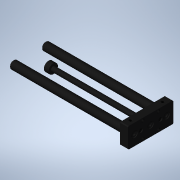
# Autodesk Inventor part: 170831 DFM-12-100-P-A-GF---(K)
Saved by Autodesk Inventor 2021 (Build 250183000, 183)
## iProperties
Created: 2025-06-15
Part Number: 170831 DFM-12-100-P-A-GF---(K)
Material: Generic
Catalog Web Link: www.cadenas.de
Description: DFM-(K)-Guide unit
Vendor: FESTO
Document SubType Name: Modeling
Designer: psAdmin
Manufacturer: FESTO
Mass: 40.9648 g
Surface Area: 173.4 cm^2
Volume: 40.9648 cm^3
Density: 1 g/cm^3
Appearance: PSOLRGB-128-128-128
Category: PARTsolutions
Company: FESTO
Title: 170831 DFM-12-100-P-A-GF---(K)
Author: Cadenas PARTsolutions
Comments: Guide unit
PSOL_IDENT_0: {$CADENAS_DATA/23d-libs/festo_fdt/parts/d/dfm/parts/dfm_k.prj},201 {VTYP=3D},{NB=170831 DFM-12-100-P
PSOL_IDENT_1: -A-GF---(K)},{LINA=170831 DFM-12-100-P-A-GF---(K)},{NN=DFM-(K)},{DATE=15.05.2025 16:58:02},{GEOMDATE=
PSOL_IDENT_2: 22.08.2023 11:13:07},{VERSION=},{LINEID=80},{WBVAR=},{WBNUMERIC=}  {NB=170831 DFM-12-100-P-A-GF---(K
PSOL_IDENT_3: )},{LINA=170831 DFM-12-100-P-A-GF---(K)},{KT=1},{TNR=170831},{TYP=DFM},{KDM=12},{HUB=100},{F=GF},{BW
PSOL_IDENT_4: E=-},{BWET=},{B4=30.000},{H1=28.000},{L8=21.000},{L9=40.000},{L11=80.000},{L7=6.000},{L1=155.000},{B
PSOL_IDENT_5: 1=60.000},{B2=58.000},{B3=42.400},{B5=4.500},{B6=51.000},{B7=20.500},{B8=19.000},{B9=20.000},{B10=20
PSOL_IDENT_6: .000},{B11=9.500},{B12=41.000},{B13=19.500},{B14=21.000},{D1=M 5},{D1P=5.000},{D1KDR=4.134},{D2=8.00
PSOL_IDENT_7: 0},{D3=9.000},{D4=M 4},{D4P=4.000},{D4KDR=3.242},{D5=0.000},{D6=M 4},{D6P=4.000},{D6KDR=3.242},{D7=1
PSOL_IDENT_8: 0},{D7GF=10.000},{D7KF=8.000},{D8=5.000},{FN=1},{FT=GF},{EE=M 5},{EEMM=5.000},{EEKDR=4.134},{H2=26.0
PSOL_IDENT_9: 00},{H3=24.000},{H4=14.000},{H5=14.000},{H6=4.000},{H7=20.000},{H8=0.000},{H9=4.000},{H10=20.000},{H
PSOL_IDENT_10: 11=14.000},{L2=136.000},{L3=10.000},{L4=13.000},{L5=11.400},{L6=9.500},{L10=34.000},{L12=11.400},{T1=
PSOL_IDENT_11: 9.000},{T2=9.400},{T3=2.100},{T4=8.000},{T5=0.000},{T6=1.000},{SW1=10.000},{SW1T=3.200},{SW2=10.000}
PSOL_IDENT_12: ,{SW2D=6.000},{SW2T=3.200},{ZZ=0},{MOD=1},{BR=8.000},{I1=25.000},{I2=41.000},{I3=4.000},{I4=8.000},{
PSOL_IDENT_13: DIML7=1},{YSCREW=0}
NB: 170831 DFM-12-100-P-A-GF---(K)
NN: DFM-(K)
NT: Guide unit
NBSYN: $TNR. $TYP.-$KDM.-$HUB.-P-A-$FT.$BWET.---(K)
LINA: 170831 DFM-12-100-P-A-GF---(K)
CATALOG: Festo Design Tool 3D
TNR: 170831
TYP: DFM
KDM: 12
HUB: 100
F: GF
BWE: -
B4: 30
H1: 28
L8: 21
L9: 40
L11: 80
L7: 6
L1: 155
B1: 60
B2: 58
B3: 42.4
B5: 4.5
B6: 51
B7: 20.5
B8: 19
B9: 20
B10: 20
B11: 9.5
B12: 41
B13: 19.5
B14: 21
D1: M 5
D1P: 5
D1KDR: 4.134
D2: 8
D3: 9
D4: M 4
D4P: 4
D4KDR: 3.242
D5: 0
D6: M 4
D6P: 4
D6KDR: 3.242
D7GF: 10
D7KF: 8
D8: 5
EE: M 5
EEKDR: 4.134
H2: 26
H3: 24
H4: 14
H5: 14
H6: 4
H7: 20
H8: 0
H9: 4
H10: 20
H11: 14
L2: 136
L3: 10
L4: 13
L5: 11.4
L6: 9.5
L10: 34
L12: 11.4
T1: 9
T2: 9.4
T3: 2.1
T4: 8
T5: 0
T6: 1
SW1: 10
SW1T: 3.2
SW2: 10
SW2D: 6
SW2T: 3.2
BR: 8
I1: 25
I2: 41
I3: 4
I4: 8
SUPPLIER: FESTO
ARTICLENO: 170831 DFM-12-100-P-A-GF---(K)
BOMINFO: 170831 DFM-12-100-P-A-GF---(K)
CREATOR: CADENAS GmbH
Autodesk Inventor part; units mm, degrees
ref_plane "YZ Plane" through (0, 0, 0) normal (1, 0, 0) x (0, 1, 0)
ref_plane "XZ Plane" through (0, 0, 0) normal (0, 1, 0) x (-1, 0, 0)
ref_plane "XY Plane" through (0, 0, 0) normal (0, 0, 1) x (1, 0, 0)
sketch "Sketch_2" plane through (13, 0, 0) normal (1, 0, 0) x (0, 0, -1)
  line L0 (-29, -12) -> (-28, -13)
  line L1 (-28, -13) -> (28, -13)
  line L2 (28, -13) -> (29, -12)
  line L3 (29, -12) -> (29, 12)
  line L4 (29, 12) -> (28, 13)
  line L5 (28, 13) -> (-28, 13)
  line L6 (-28, 13) -> (-29, 12)
  line L7 (-29, 12) -> (-29, -12)
  constraints: 16 end point
sketch "Sketch_3" plane through (0, 0, 0) normal (0, 1, 0) x (1, 0, 0)
  line L0 (13, 20.5) -> (-142, 20.5)
  line L1 (-142, 20.5) -> (-142, 24.5)
  line L2 (-142, 24.5) -> (-141, 25.5)
  line L3 (-141, 25.5) -> (13, 25.5)
  line L4 (13, 25.5) -> (13, 20.5)
  line L5 (13, 20.5) -> (-142, 20.5)
  constraints: 12 end point
sketch "Sketch_4" plane through (0, 0, 0) normal (0, 1, 0) x (1, 0, 0)
  line L0 (13, -20.5) -> (-142, -20.5)
  line L1 (-142, -20.5) -> (-142, -16.5)
  line L2 (-142, -16.5) -> (-141, -15.5)
  line L3 (-141, -15.5) -> (13, -15.5)
  line L4 (13, -15.5) -> (13, -20.5)
  line L5 (13, -20.5) -> (-142, -20.5)
  constraints: 12 end point
extrude "Extrusion1" add sketch "Sketch_2" against normal blind 10
sketch "Sketch_8" plane through (0, 10, 0) normal (0, 1, 0) x (1, 0, 0)
  line L0 (13, 10) -> (3, 10)
  line L1 (3, 10) -> (3, 12)
  line L2 (3, 12) -> (3.379, 11.621)
  line L3 (3.379, 11.621) -> (12.621, 11.621)
  line L4 (12.621, 11.621) -> (13, 12)
  line L5 (13, 12) -> (13, 10)
  line L6 (13, 10) -> (3, 10)
  constraints: 14 end point
revolve "Revolution1" cut sketch "Sketch_8" angle 360 about axis through (13, 10, -10) along (-1, 0, 0)
thread "Thread1" size "M4x0.7" class "6H" standard "ISO Metric profile" full length
sketch "Sketch_9" plane through (0, 10, 0) normal (0, 1, 0) x (1, 0, 0)
  line L0 (13, -10) -> (3, -10)
  line L1 (3, -10) -> (3, -8)
  line L2 (3, -8) -> (3.379, -8.379)
  line L3 (3.379, -8.379) -> (12.621, -8.379)
  line L4 (12.621, -8.379) -> (13, -8)
  line L5 (13, -8) -> (13, -10)
  line L6 (13, -10) -> (3, -10)
  constraints: 14 end point
revolve "Revolution2" cut sketch "Sketch_9" angle 360 about axis through (13, 10, 10) along (-1, 0, 0)
thread "Thread2" size "M4x0.7" class "6H" standard "ISO Metric profile" full length
sketch "Sketch_12" plane through (0, -10, 0) normal (0, 1, 0) x (1, 0, 0)
  line L0 (13, 10) -> (3, 10)
  line L1 (3, 10) -> (3, 12)
  line L2 (3, 12) -> (3.379, 11.621)
  line L3 (3.379, 11.621) -> (12.621, 11.621)
  line L4 (12.621, 11.621) -> (13, 12)
  line L5 (13, 12) -> (13, 10)
  line L6 (13, 10) -> (3, 10)
  constraints: 14 end point
revolve "Revolution3" cut sketch "Sketch_12" angle 360 about axis through (13, -10, -10) along (-1, 0, 0)
thread "Thread3" size "M4x0.7" class "6H" standard "ISO Metric profile" full length
sketch "Sketch_13" plane through (0, -10, 0) normal (0, 1, 0) x (1, 0, 0)
  line L0 (13, -10) -> (3, -10)
  line L1 (3, -10) -> (3, -8)
  line L2 (3, -8) -> (3.379, -8.379)
  line L3 (3.379, -8.379) -> (12.621, -8.379)
  line L4 (12.621, -8.379) -> (13, -8)
  line L5 (13, -8) -> (13, -10)
  line L6 (13, -10) -> (3, -10)
  constraints: 14 end point
revolve "Revolution4" cut sketch "Sketch_13" angle 360 about axis through (13, -10, 10) along (-1, 0, 0)
thread "Thread4" size "M4x0.7" class "6H" standard "ISO Metric profile" full length
sketch "Skizze_3" plane through (0, 0, 0) normal (0, 0, 1) x (1, 0, 0)
  line L0 (3, 0) -> (-117.4, 0)
  line L1 (-117.4, 0) -> (-117.4, 6)
  line L2 (-117.4, 6) -> (-111.4, 6)
  line L3 (-111.4, 6) -> (-111.4, 3)
  line L4 (-111.4, 3) -> (3, 3)
  line L5 (3, 3) -> (3, 0)
  line L6 (3, 0) -> (-117.4, 0)
  constraints: 14 end point
revolve "Revolution5" add sketch "Skizze_3" angle 360 about axis through (3, 0, 0) along (-1, 0, 0)
sketch "Sketch_17" plane through (0, 0, 0) normal (1, 0, 0) x (0, 1, 0)
  line L0 (-10, 7.5) -> (-10, -7.5)
  line L1 (-10, -7.5) -> (10, -7.5)
  line L2 (10, -7.5) -> (10, 7.5)
  line L3 (10, 7.5) -> (-10, 7.5)
  line L4 (-5, 2.75) -> (-5, -2.75)
  line L5 (-5, -2.75) -> (5, -2.75)
  line L6 (5, -2.75) -> (5, 2.75)
  line L7 (5, 2.75) -> (-5, 2.75)
  constraints: 16 end point
extrude "Extrusion2" cut sketch "Sketch_17" along normal blind 3
sketch "Sketch10" plane through (13, 0, 0) normal (1, 0, 0) x (0, 0, -1)
  point P0 (12.5, 0)
hole "Hole1" at (13, 0, -12.5) direction (-1, 0, 0) diameter 5 depth 1.2 tip angle 120
sketch "Sketch11" plane through (13, 0, 0) normal (1, 0, 0) x (0, 0, -1)
  point P0 (-12.5, 0)
hole "Hole2" at (13, 0, 12.5) direction (-1, 0, 0) diameter 5 depth 1.2 tip angle 120
sketch "Sketch12" plane through (13, 13, 28) normal (0, 1, 0) x (1, 0, 0)
  point P0 (-5, 48.5)
hole "Hole3" at (8, 13, -20.5) direction (0, -1, 0) diameter 3.242 depth 13 countersink diameter 4 countersink angle 90 thread size "M4x0.7" class "6H" standard "ISO Metric profile"
sketch "Sketch13" plane through (13, 13, 28) normal (0, 1, 0) x (1, 0, 0)
  point P0 (-5, 7.5)
hole "Hole4" at (8, 13, 20.5) direction (0, -1, 0) diameter 3.242 depth 13 countersink diameter 4 countersink angle 90 thread size "M4x0.7" class "6H" standard "ISO Metric profile"
revolve "Revolution6" add sketch "Sketch_4" angle 360 about axis through (13, 0, 20.5) along (1, 0, 0)
revolve "Revolution7" add sketch "Sketch_3" angle 360 about axis through (13, 0, -20.5) along (1, 0, 0)
sketch "Sketch_20" plane through (13, 0, 0) normal (1, 0, 0) x (0, 0, -1)
  arc A0 (-1.6342, -0.5011) -> (-1.2511, -1.1647) centre (-1.364, -0.7875) ccw
  arc A1 (-0.3831, -1.6659) -> (-1.2511, -1.1647) centre (-1.0536, -1.8249) ccw
  arc A2 (-0.3831, -1.6659) -> (0.3831, -1.6659) centre (0, -1.575) ccw
  arc A3 (1.2511, -1.1647) -> (0.3831, -1.6659) centre (1.0536, -1.8249) ccw
  arc A4 (1.2511, -1.1647) -> (1.6342, -0.5011) centre (1.364, -0.7875) ccw
  arc A5 (1.6342, 0.5011) -> (1.6342, -0.5011) centre (2.1072, 0) ccw
  arc A6 (1.6342, 0.5011) -> (1.2511, 1.1647) centre (1.364, 0.7875) ccw
  arc A7 (0.3831, 1.6659) -> (1.2511, 1.1647) centre (1.0536, 1.8249) ccw
  arc A8 (0.3831, 1.6659) -> (-0.3831, 1.6659) centre (0, 1.575) ccw
  arc A9 (-1.2511, 1.1647) -> (-0.3831, 1.6659) centre (-1.0536, 1.8249) ccw
  arc A10 (-1.2511, 1.1647) -> (-1.6342, 0.5011) centre (-1.364, 0.7875) ccw
  arc A11 (-1.6342, -0.5011) -> (-1.6342, 0.5011) centre (-2.1072, 0) ccw
  constraints: 24 point on circle, 12 centre point
extrude "Extrusion3" cut sketch "Sketch_20" against normal blind 2
sketch "Pattern_2_SKETCH_1" plane through (13, 0, 0) normal (1, 0, 0) x (0, 0, -1)
  arc A0 (18.8658, -0.5011) -> (19.2489, -1.1647) centre (19.136, -0.7875) ccw
  arc A1 (20.1169, -1.6659) -> (19.2489, -1.1647) centre (19.4464, -1.8249) ccw
  arc A2 (20.1169, -1.6659) -> (20.8831, -1.6659) centre (20.5, -1.575) ccw
  arc A3 (21.7511, -1.1647) -> (20.8831, -1.6659) centre (21.5536, -1.8249) ccw
  arc A4 (21.7511, -1.1647) -> (22.1342, -0.5011) centre (21.864, -0.7875) ccw
  arc A5 (22.1342, 0.5011) -> (22.1342, -0.5011) centre (22.6072, 0) ccw
  arc A6 (22.1342, 0.5011) -> (21.7511, 1.1647) centre (21.864, 0.7875) ccw
  arc A7 (20.8831, 1.6659) -> (21.7511, 1.1647) centre (21.5536, 1.8249) ccw
  arc A8 (20.8831, 1.6659) -> (20.1169, 1.6659) centre (20.5, 1.575) ccw
  arc A9 (19.2489, 1.1647) -> (20.1169, 1.6659) centre (19.4464, 1.8249) ccw
  arc A10 (19.2489, 1.1647) -> (18.8658, 0.5011) centre (19.136, 0.7875) ccw
  arc A11 (18.8658, -0.5011) -> (18.8658, 0.5011) centre (18.3928, 0) ccw
  constraints: 24 point on circle, 12 centre point
sketch "Pattern_2_SKETCH_2" plane through (13, 0, 0) normal (1, 0, 0) x (0, 0, -1)
  arc A0 (-22.1342, -0.5011) -> (-21.7511, -1.1647) centre (-21.864, -0.7875) ccw
  arc A1 (-20.8831, -1.6659) -> (-21.7511, -1.1647) centre (-21.5536, -1.8249) ccw
  arc A2 (-20.8831, -1.6659) -> (-20.1169, -1.6659) centre (-20.5, -1.575) ccw
  arc A3 (-19.2489, -1.1647) -> (-20.1169, -1.6659) centre (-19.4464, -1.8249) ccw
  arc A4 (-19.2489, -1.1647) -> (-18.8658, -0.5011) centre (-19.136, -0.7875) ccw
  arc A5 (-18.8658, 0.5011) -> (-18.8658, -0.5011) centre (-18.3928, 0) ccw
  arc A6 (-18.8658, 0.5011) -> (-19.2489, 1.1647) centre (-19.136, 0.7875) ccw
  arc A7 (-20.1169, 1.6659) -> (-19.2489, 1.1647) centre (-19.4464, 1.8249) ccw
  arc A8 (-20.1169, 1.6659) -> (-20.8831, 1.6659) centre (-20.5, 1.575) ccw
  arc A9 (-21.7511, 1.1647) -> (-20.8831, 1.6659) centre (-21.5536, 1.8249) ccw
  arc A10 (-21.7511, 1.1647) -> (-22.1342, 0.5011) centre (-21.864, 0.7875) ccw
  arc A11 (-22.1342, -0.5011) -> (-22.1342, 0.5011) centre (-22.6072, 0) ccw
  constraints: 24 point on circle, 12 centre point
extrude "Extrusion4" cut sketch "Pattern_2_SKETCH_1" against normal blind 2
extrude "Extrusion5" cut sketch "Pattern_2_SKETCH_2" against normal blind 2
sketch "Sketch_22" plane through (0, 0, 0) normal (0, 1, 0) x (1, 0, 0)
  line L0 (13, 0) -> (12.6, 0)
  line L1 (12.6, 0) -> (12.6, 3)
  arc A0 (12.6, 3) -> (12.1, 3.5) centre (12.1, 3) ccw
  line L2 (12.1, 3.5) -> (9.5, 3.5)
  line L3 (9.5, 3.5) -> (9.5, 4)
  line L4 (9.5, 4) -> (13, 4)
  line L5 (13, 4) -> (13, 0)
  line L6 (13, 0) -> (12.6, 0)
  constraints: 14 end point, 2 point on circle, 1 centre point
revolve "Revolution8" cut sketch "Sketch_22" angle 360 about axis through (13, 0, 0) along (-1, 0, 0)
sketch "Pattern_3_SKETCH_1" plane through (0, 0, 20.5) normal (0, 1, 0) x (1, 0, 0)
  line L0 (13, 0) -> (12.6, 0)
  line L1 (12.6, 0) -> (12.6, 3)
  arc A0 (12.6, 3) -> (12.1, 3.5) centre (12.1, 3) ccw
  line L2 (12.1, 3.5) -> (9.5, 3.5)
  line L3 (9.5, 3.5) -> (9.5, 4)
  line L4 (9.5, 4) -> (13, 4)
  line L5 (13, 4) -> (13, 0)
  line L6 (13, 0) -> (12.6, 0)
  constraints: 14 end point, 2 point on circle, 1 centre point
sketch "Pattern_3_SKETCH_2" plane through (0, 0, -20.5) normal (0, 1, 0) x (1, 0, 0)
  line L0 (13, 0) -> (12.6, 0)
  line L1 (12.6, 0) -> (12.6, 3)
  arc A0 (12.6, 3) -> (12.1, 3.5) centre (12.1, 3) ccw
  line L2 (12.1, 3.5) -> (9.5, 3.5)
  line L3 (9.5, 3.5) -> (9.5, 4)
  line L4 (9.5, 4) -> (13, 4)
  line L5 (13, 4) -> (13, 0)
  line L6 (13, 0) -> (12.6, 0)
  constraints: 14 end point, 2 point on circle, 1 centre point
revolve "Revolution9" cut sketch "Pattern_3_SKETCH_1" angle 360 about axis through (13, 0, 20.5) along (-1, 0, 0)
revolve "Revolution10" cut sketch "Pattern_3_SKETCH_2" angle 360 about axis through (13, 0, -20.5) along (-1, 0, 0)
ref_plane "HUELSE3_1_XY" through (11.8, 0, -12.5) normal (1, 0, 0) x (0, 0, -1)
ref_plane "HUELSE3_1_YZ" through (11.8, 0, -12.5) normal (0, 0, -1) x (0, 1, 0)
ref_plane "HUELSE3_1_ZX" through (11.8, 0, -12.5) normal (0, 1, 0) x (1, 0, 0)
ref_plane "HUELSE3_2_XY" through (11.8, 0, 12.5) normal (1, 0, 0) x (0, 0, -1)
ref_plane "HUELSE3_2_YZ" through (11.8, 0, 12.5) normal (0, 0, -1) x (0, 1, 0)
ref_plane "HUELSE3_2_ZX" through (11.8, 0, 12.5) normal (0, 1, 0) x (1, 0, 0)
ref_plane "dfm_k_XY" through (0, 0, 0) normal (-1, 0, 0) x (0, 0, -1)
ref_plane "dfm_k_YZ" through (0, 0, 0) normal (0, 0, -1) x (0, -1, 0)
ref_plane "dfm_k_ZX" through (0, 0, 0) normal (0, -1, 0) x (-1, 0, 0)
body "Solid1"
